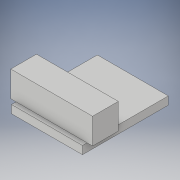
# Autodesk Inventor part: ShockSensor
Saved by Autodesk Inventor 2017 (Build 210142000, 142)
## iProperties
Created: 2018-12-12
Part Number: ShockSensor
Material: Generic
Document SubType Name: Modeling
Designer: S346795925
Density: 1 g/cm^3
Appearance: Default
Author: S346795925
Autodesk Inventor part; units mm, degrees
ref_plane "YZ Plane" through (0, 0, 0) normal (1, 0, 0) x (0, 1, 0)
ref_plane "XZ Plane" through (0, 0, 0) normal (0, 1, 0) x (-1, 0, 0)
ref_plane "XY Plane" through (0, 0, 0) normal (0, 0, 1) x (1, 0, 0)
sketch "Sketch1" plane through (0, 0, 0) normal (0, 1, 0) x (-1, 0, 0)
  line L0 (0, 0) -> (-15.748, 0)
  line L1 (-15.748, 0) -> (-15.748, -19.05)
  line L2 (-15.748, -19.05) -> (0, -19.05)
  line L3 (0, -19.05) -> (0, 0)
  dimension "d0" = 15.748
  dimension "d1" = 19.05
  constraints: 8 end point, 2 parallel, 1 horizontal, 1 perpendicular
  measures "d0" distance of L2.end L1.end
  measures "d1" distance of L1.end L0.end
extrude "Extrusion1" add sketch "Sketch1" along normal blind 1.778
sketch "Sketch2" plane through (0, 1.778, 0) normal (0, 1, 0) x (1, 0, 0)
  line L0 (0, 0) -> (15.748, 0) projected
  line L1 (15.748, 0) -> (15.748, 19.05) projected
  line L2 (15.748, 19.05) -> (0, 19.05) projected
  line L3 (0, 19.05) -> (0, 0) projected
  line L4 (0, 19.05) -> (0, 0) projected
  line L5 (-1.1891, 1.016) -> (16.9719, 1.016)
  line L6 (-1.1891, 6.731) -> (16.9719, 6.731)
  line L7 (-1.1891, 1.016) -> (-1.1891, 6.731)
  line L8 (16.9719, 1.016) -> (16.9719, 6.731)
  dimension "d4" = 1.016
  dimension "d5" = 5.715
  dimension "d6" = 18.161
  constraints: 8 end point, 3 vertical, 1 parallel, 1 perpendicular
  measures "d4" distance between parallel lines of L0 L5
  measures "d5" distance between parallel lines of L5 L6
  measures "d6" distance between parallel lines of L8 L7
extrude "Extrusion2" add sketch "Sketch2" along normal blind 5.715 contours L5 L7 L6 L3 | L3 L6 L1 L5 | L1 L6 L8 L5
body "Solid1"
